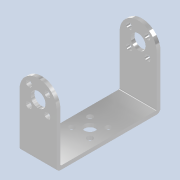
# Autodesk Inventor part: サーボモーター25kgcmサーボホーン2
Saved by Autodesk Inventor 2021.2 (Build 252289000, 289)
## iProperties
Created: 2020-02-02
Part Number: サーボモーター25kgcmサーボホーン2
Material: アルミニウム 6061
Document SubType Name: Modeling
Designer: yuta2
Density: 2.7 g/cm^3
Appearance: アルミニウム - フラット
Author: yuta2
Autodesk Inventor part; units mm, degrees
ref_plane "YZ Plane" through (0, 0, 0) normal (1, 0, 0) x (0, 1, 0)
ref_plane "XZ Plane" through (0, 0, 0) normal (0, 1, 0) x (-1, 0, 0)
ref_plane "XY Plane" through (0, 0, 0) normal (0, 0, 1) x (1, 0, 0)
sketch "スケッチ1" plane through (0, 0, 0) normal (1, 0, 0) x (0, 1, 0)
  line L0 (0, 0) -> (2, 0)
  line L1 (2, 0) -> (2, -56)
  line L2 (2, -56) -> (0, -56)
  line L3 (0, -56) -> (0, 0)
  line L4 (2, 0) -> (39, 0)
  line L5 (39, 0) -> (39, -2)
  line L6 (39, -2) -> (2, -2)
  line L7 (2, -2) -> (2, 0)
  line L8 (2, -56) -> (39, -56)
  line L9 (39, -56) -> (39, -54)
  line L10 (39, -54) -> (2, -54)
  line L11 (2, -54) -> (2, -56)
  point P0 (2, -54)
  point P1 (2, -2)
  dimension "d0" = 2
  dimension "d1" = 56
  dimension "d2" = 37
  dimension "d3" = 2
  dimension "d4" = 37
  dimension "d5" = 2
  constraints: 24 end point, 6 parallel, 3 horizontal, 3 perpendicular
  measures "d0" distance of L1.end L2.end
  measures "d1" distance of L0.end L1.end
  measures "d2" distance of L5.end L6.end
  measures "d3" distance of L4.end L5.end
  measures "d4" distance of L10.end L9.end
  measures "d5" distance of L9.end L8.end
extrude "押し出し1" add sketch "スケッチ1" along normal blind 20
sketch "スケッチ2" plane through (0, 0, 0) normal (0, 0, 1) x (1, 0, 0)
  arc A0 (20, 29) -> (0, 29) centre (10, 29) ccw
  line L0 (0, 39) -> (20, 39) projected
  line L1 (0, 39) -> (0, 0) projected
  line L2 (20, 39) -> (20, 0) projected
  point P0 (10, 39)
  dimension "d8" = 10
  constraints: 2 point on circle, 2 point on line, 2 tangent, 1 centre point
  measures "d8" radius of A0
extrude "押し出し2" cut sketch "スケッチ2" against normal through all
sketch "スケッチ3" plane through (0, 0, 0) normal (0, 0, 1) x (1, 0, 0)
  arc A0 (20, 29) -> (0, 29) centre (10, 29) ccw projected
  point P0 (0, 0)
  point P1 (5, 34)
  point P2 (15, 34)
  point P3 (15, 24)
  point P4 (5, 24)
  dimension "d11" = 5
  dimension "d12" = 5
  dimension "d13" = 10
  dimension "d14" = 10
  constraints: 2 horizontal alignment, 2 vertical alignment
  measures "d11" horizontal distance of A0.centre point (5, 34)
  measures "d12" horizontal distance of A0.centre point (5, 34)
  measures "d13" distance of point (15, 34) point (5, 34)
  measures "d14" distance of point (15, 34) point (15, 24)
hole "穴1" at (5, 34, 0) at (15, 34, 0) at (15, 24, 0) at (5, 24, 0) direction (0, 0, -1) diameter 3.2 end through all
sketch "スケッチ4" plane through (0, 0, 0) normal (0, 0, 1) x (1, 0, 0)
  arc A0 (20, 29) -> (0, 29) centre (10, 29) ccw projected
  circle A1 centre (10, 29) radius 4
  point P0 (0, 0)
  dimension "d22" = 8
  constraints: 1 centre point, 1 coincident
  measures "d22" diameter of A1
extrude "押し出し3" cut sketch "スケッチ4" against normal through all
fillet "フィレット1" radius 0.5 2 edges at (10, 2, -54) (10, 2, -2)
fillet "フィレット2" radius 2 2 edges at (10, 0, -56) (10, 0, 0)
sketch "スケッチ5" plane through (0, 2, -2.5) normal (0, 1, 0) x (1, 0, 0)
  line L0 (0, -0.5) -> (0, 51.5) projected
  line L1 (0, 25.5) -> (20, 25.5)
  line L2 (20, 51) -> (20, 0) projected
  line L3 (20, 51.5) -> (0, 51.5) projected
  line L4 (10, 51.5) -> (10, 0)
  line L5 (20, 0) -> (0, 0) projected
  point P0 (0, -2.5)
  point P1 (5, 30.5)
  point P2 (15, 30.5)
  point P3 (15, 20.5)
  point P4 (5, 20.5)
  dimension "d27" = 10
  dimension "d28" = 10
  constraints: 4 end point, 4 midpoint, 3 symmetric about line
  measures "d27" distance of point (15, 20.5) point (5, 20.5)
  measures "d28" distance of point (15, 20.5) point (15, 30.5)
hole "穴2" at (5, 2, -33) at (15, 2, -33) at (15, 2, -23) at (5, 2, -23) direction (0, -1, 0) diameter 3.2 end through all
sketch "スケッチ6" plane through (0, 2, -2.5) normal (0, 1, 0) x (1, 0, 0)
  circle A0 centre (10, 25.5) radius 3
  circle A1 centre (5, 20.5) radius 1.6 projected
  point P0 (0, -2.5)
  dimension "d36" = 6
  dimension "d37" = 5
  dimension "d38" = 5
  constraints: 1 centre point
  measures "d36" diameter of A0
  measures "d37" horizontal distance of A1.centre A0.centre
  measures "d38" horizontal distance of A0.centre A1.centre
extrude "押し出し4" cut sketch "スケッチ6" against normal through all contours A0
